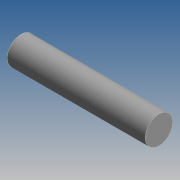
# Autodesk Inventor part: M002
Saved by Autodesk Inventor 2017 (Build 210142000, 142)
## iProperties
Created: 2018-10-19
Part Number: M002
Material: Acier / Stahl
Document SubType Name: Modeling
Designer: Gilles Mottiez
Density: 7.85 g/cm^3
Appearance: Par défaut
Description: Goupille de maintien du ressort
Author: Gilles Mottiez
Autodesk Inventor part; units mm, degrees
ref_plane "YZ Plane" through (0, 0, 0) normal (1, 0, 0) x (0, 1, 0)
ref_plane "XZ Plane" through (0, 0, 0) normal (0, 1, 0) x (-1, 0, 0)
ref_plane "XY Plane" through (0, 0, 0) normal (0, 0, 1) x (1, 0, 0)
sketch "Sketch1" plane through (0, 0, 0) normal (0, 0, 1) x (1, 0, 0)
  line L0 (0, 0) -> (15, 0)
  line L1 (0, 0) -> (0, 1.5)
  line L2 (0, 1.5) -> (15, 1.5)
  line L3 (15, 1.5) -> (15, 0)
  dimension "d0" = 15
  dimension "d2" = 3
  constraints: 8 end point, 2 perpendicular, 1 horizontal, 1 vertical
  measures "d0" distance of L0.start L0.end
  measures "d2" diameter of L2 L0
revolve "Révolution1" add sketch "Sketch1" angle 360 about axis through (0, 0, 0) along (1, 0, 0)
